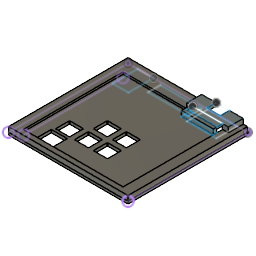
Aiwa up (Autodesk Fusion 360 design; units mm, degrees)
part number: 2026-08-31-21-16-21-827
Autodesk Fusion 360 part; units mm, degrees
note: some values were not read from the file. Chosen so that the rebuilt part matches the saved one: which bodies a step acts on. Set by a fixed rule: which sketch regions a step uses.
sketch "Sketch1" plane through (0, 0, 0) normal (0, 0, 1) x (1, 0, 0)
  line L0 (-50, 42.3306) -> (50, 42.3306)
  line L1 (50, 42.3306) -> (50, -57.6694)
  line L2 (50, -57.6694) -> (-50, -57.6694)
  line L3 (-50, -57.6694) -> (-50, 42.3306)
  line L4 (-60, 57.3306) -> (60, 57.3306)
  line L5 (60, 57.3306) -> (60, -62.6694)
  line L6 (60, -62.6694) -> (-60, -62.6694)
  line L7 (-60, -62.6694) -> (-60, 57.3306)
  dimension "d1" = 120
  dimension "d2" = 120
  dimension "d3" = 5
  dimension "d4" = 10
  dimension "d5" = 10
  dimension "d6" = 15
  constraint horizontal L0
  constraint vertical L1
  constraint horizontal L2
  constraint vertical L3
  constraint horizontal L4
  constraint vertical L5
  constraint horizontal L6
  constraint vertical L7
  measures "d1" distance of L4.start L4.end
  measures "d2" distance of L4.start L6.end
  measures "d3" distance of L2 L6
  measures "d4" distance of L3 L7
  measures "d5" distance of L1 L5
  measures "d6" distance of L0 L4
extrude "Extrude1" add sketch "Sketch1" along normal blind 3 contours L0 L1 L2 L3 makes body 1
extrude "Extrude2" add sketch "Sketch1" along normal blind 5 bodies 1
sketch "Sketch2" plane through (0, 0, 0) normal (0, 0, 1) x (1, 0, 0)
  line L0 (16.456, 54.7196) -> (-24.775, 54.7196)
  line L1 (-24.775, 54.7196) -> (-24.775, 42.3306)
  line L2 (-24.775, 42.3306) -> (16.456, 42.3306)
  line L3 (16.456, 42.3306) -> (16.456, 54.7196)
  line L4 (-60, 57.3306) -> (60, 57.3306)
  line L5 (-60, -62.6694) -> (-60, 57.3306)
  line L6 (60, 57.3306) -> (60, -62.6694)
  line L7 (-34.3292, 57.3306) -> (-50.3292, 57.3306)
  line L8 (-50.3292, 57.3306) -> (-50.3292, 32.0777)
  line L9 (-50.3292, 32.0777) -> (-34.3292, 32.0777)
  line L10 (-34.3292, 32.0777) -> (-34.3292, 57.3306)
  line L11 (-50, -57.6694) -> (-50, 42.3306)
  line L12 (20.1, 36.3376) -> (49.6, 36.3376)
  line L13 (49.6, 36.3376) -> (49.6, 57.3376)
  line L14 (49.6, 57.3376) -> (20.1, 57.3376)
  line L15 (20.1, 57.3376) -> (20.1, 36.3376)
  dimension "d11" = 41.231
  dimension "d12" = 12.389
  dimension "d14" = 35.225
  dimension "d15" = 43.544
  dimension "d18" = 16
  dimension "d72" = 29.5
  dimension "d73" = 21
  dimension "d74" = 10
  dimension "d75" = 10.4
  constraint horizontal L0
  constraint vertical L1
  constraint horizontal L2
  constraint vertical L3
  constraint horizontal L7
  constraint vertical L8
  constraint horizontal L9
  constraint vertical L10
  constraint coincident L4 L7.start
  constraint horizontal L12
  constraint vertical L13
  constraint horizontal L14
  constraint vertical L15
  measures "d11" distance of L0.start L0.end
  measures "d12" distance of L0.start L2.end
  measures "d14" distance of L1 L5
  measures "d15" distance of L3 L6
  measures "d18" distance of L7.start L7.end
  measures "d72" distance of L12.start L12.end
  measures "d73" distance of L12.start L14.end
  measures "d74" distance of L5 L11
  measures "d75" distance of L6 L13
surface "Extrude3" add extruded along (0, 0, 1) between 0 and 1.5 profiles "Sketch2" section 1 contours L4 L7 L8 L9 L10 separate body makes body 2
extrude "Extrude4" cut sketch "Sketch2" along normal blind 2.5 contours L0 L1 L2 L3 bodies 1
sketch "Sketch3" plane through (0, 0, 5) normal (0, 0, 1) x (-1, 0, 0)
  line L0 (-50, 57.6694) -> (50, 57.6694)
  line L1 (50, 57.6694) -> (50, -42.3306)
  line L2 (50, -42.3306) -> (-50, -42.3306)
  line L3 (-50, -42.3306) -> (-50, 57.6694)
  line L4 (60, 62.6694) -> (-60, 62.6694)
  line L5 (-60, 62.6694) -> (-60, -57.3306)
  line L6 (-60, -57.3306) -> (60, -57.3306)
  line L7 (60, -57.3306) -> (60, 62.6694)
  line L8 (-13.9272, -57.3306) -> (-55.7769, -57.3306)
  line L9 (-55.7769, -57.3306) -> (-55.7769, -42.3306)
  line L10 (-55.7769, -42.3306) -> (-13.9272, -42.3306)
  line L11 (-13.9272, -42.3306) -> (-13.9272, -57.3306)
  dimension "d80" = 15
  constraint horizontal L8
  constraint vertical L9
  constraint horizontal L10
  constraint vertical L11
  constraint coincident L2 L9.end
  constraint coincident L6 L8.start
  measures "d80" distance of L8.start L10.end
extrude "Extrude5" add sketch "Sketch3" along normal blind 5 contours L2 L6 L8 L9 L10 L11 bodies 1
extrude "Extrude6" cut sketch "Sketch2" along normal blind 7 contours L4 L12 L13 L15 bodies 1
extrude "Extrude7" add sketch "Sketch1" against normal blind 2.5 separate body makes body 3
extrude "Extrude8" cut sketch "Sketch2" against normal blind 2.5 contours L4 L12 L13 L15 bodies 3
extrude "Extrude9" cut sketch "Sketch2" against normal blind 2.5 contours L0 L1 L2 L3 bodies 3
extrude "Extrude10" cut sketch "Sketch2" against normal blind 2.5 contours L4 L7 L8 L9 L10 bodies 3 makes body 4 at (56.6667, 12.3306, 0)
sketch "Sketch4" plane through (0, 0, 0) normal (0, 0, 1) x (1, 0, 0)
  line L0 (38, -41.6694) -> (22, -41.6694)
  line L1 (22, -41.6694) -> (22, -56.1694)
  line L2 (22, -56.1694) -> (38, -56.1694)
  line L3 (38, -56.1694) -> (38, -41.6694)
  line L4 (50, -57.6694) -> (-50, -57.6694)
  line L5 (50, 42.3306) -> (50, -57.6694)
  dimension "d37" = 16
  dimension "d38" = 14.5
  dimension "d39" = 1.5
  dimension "d40" = 12
  constraint horizontal L0
  constraint vertical L1
  constraint horizontal L2
  constraint vertical L3
  measures "d37" distance of L0.start L0.end
  measures "d38" distance of L0.start L2.end
  measures "d39" distance of L2 L4
  measures "d40" distance of L3 L5
extrude "Extrude11" cut sketch "Sketch4" along normal blind 3 bodies 1
sketch "Sketch5" plane through (0, 0, 0) normal (0, 0, -1) x (1, 0, 0)
  line L0 (22, 56.1694) -> (38, 56.1694)
  line L1 (38, 56.1694) -> (38, 41.6694)
  line L2 (38, 41.6694) -> (22, 41.6694)
  line L3 (22, 41.6694) -> (22, 56.1694)
  line L4 (49.6, -57.3306) -> (60, -57.3306)
  line L5 (60, -57.3306) -> (60, 62.6694)
  line L6 (60, 62.6694) -> (-60, 62.6694)
  line L7 (-60, 62.6694) -> (-60, -57.3306)
  line L8 (-60, -57.3306) -> (20.1, -57.3306)
  line L9 (-24.775, -42.3306) -> (16.456, -42.3306)
  line L10 (16.456, -42.3306) -> (16.456, -54.7196)
  line L11 (16.456, -54.7196) -> (-24.775, -54.7196)
  line L12 (-24.775, -54.7196) -> (-24.775, -42.3306)
  line L13 (18.153, 22.4292) -> (-0.897, 22.4292)
  line L14 (-0.897, 22.4292) -> (-0.897, 41.4792)
  line L15 (-0.897, 41.4792) -> (18.153, 41.4792)
  line L16 (18.153, 41.4792) -> (18.153, 22.4292)
  line L17 (50, -42.3306) -> (50, 57.6694)
  line L18 (2.0861, 38.928) -> (15.0861, 38.928)
  line L19 (2.0861, 24.928) -> (15.0861, 24.928)
  line L20 (1.5861, 38.428) -> (1.5861, 25.428)
  line L21 (15.5861, 38.428) -> (15.5861, 25.428)
  arc A0 (2.0861, 38.928) -> (1.5861, 38.428) centre (2.0861, 38.428) ccw
  arc A1 (15.5861, 38.428) -> (15.0861, 38.928) centre (15.0861, 38.428) ccw
  arc A2 (1.5861, 25.428) -> (2.0861, 24.928) centre (2.0861, 25.428) ccw
  arc A3 (15.0861, 24.928) -> (15.5861, 25.428) centre (15.0861, 25.428) ccw
  line L22 (-0.9389, 22.403) -> (18.1111, 22.403)
  line L23 (-0.9389, 41.453) -> (18.1111, 41.453)
  line L24 (-0.9389, 22.403) -> (-0.9389, 41.453)
  line L25 (18.1111, 22.403) -> (18.1111, 41.453)
  line L26 (-16.9175, 38.9647) -> (-3.9175, 38.9647)
  line L27 (-16.9175, 24.9647) -> (-3.9175, 24.9647)
  line L28 (-17.4175, 38.4647) -> (-17.4175, 25.4647)
  line L29 (-3.4175, 38.4647) -> (-3.4175, 25.4647)
  arc A4 (-16.9175, 38.9647) -> (-17.4175, 38.4647) centre (-16.9175, 38.4647) ccw
  arc A5 (-3.4175, 38.4647) -> (-3.9175, 38.9647) centre (-3.9175, 38.4647) ccw
  arc A6 (-17.4175, 25.4647) -> (-16.9175, 24.9647) centre (-16.9175, 25.4647) ccw
  arc A7 (-3.9175, 24.9647) -> (-3.4175, 25.4647) centre (-3.9175, 25.4647) ccw
  line L30 (-19.9425, 22.4397) -> (-0.8925, 22.4397)
  line L31 (-19.9425, 41.4897) -> (-0.8925, 41.4897)
  line L32 (-19.9425, 22.4397) -> (-19.9425, 41.4897)
  line L33 (-0.8925, 22.4397) -> (-0.8925, 41.4897)
  line L34 (-35.9551, 38.9464) -> (-22.9551, 38.9464)
  line L35 (-35.9551, 24.9464) -> (-22.9551, 24.9464)
  line L36 (-36.4551, 38.4464) -> (-36.4551, 25.4464)
  line L37 (-22.4551, 38.4464) -> (-22.4551, 25.4464)
  arc A8 (-35.9551, 38.9464) -> (-36.4551, 38.4464) centre (-35.9551, 38.4464) ccw
  arc A9 (-22.4551, 38.4464) -> (-22.9551, 38.9464) centre (-22.9551, 38.4464) ccw
  arc A10 (-36.4551, 25.4464) -> (-35.9551, 24.9464) centre (-35.9551, 25.4464) ccw
  arc A11 (-22.9551, 24.9464) -> (-22.4551, 25.4464) centre (-22.9551, 25.4464) ccw
  line L38 (-38.9801, 22.4214) -> (-19.9301, 22.4214)
  line L39 (-38.9801, 41.4714) -> (-19.9301, 41.4714)
  line L40 (-38.9801, 22.4214) -> (-38.9801, 41.4714)
  line L41 (-19.9301, 22.4214) -> (-19.9301, 41.4714)
  line L42 (2.0843, 19.8957) -> (15.0843, 19.8957)
  line L43 (2.0843, 5.8957) -> (15.0843, 5.8957)
  line L44 (1.5843, 19.3957) -> (1.5843, 6.3957)
  line L45 (15.5843, 19.3957) -> (15.5843, 6.3957)
  arc A12 (2.0843, 19.8957) -> (1.5843, 19.3957) centre (2.0843, 19.3957) ccw
  arc A13 (15.5843, 19.3957) -> (15.0843, 19.8957) centre (15.0843, 19.3957) ccw
  arc A14 (1.5843, 6.3957) -> (2.0843, 5.8957) centre (2.0843, 6.3957) ccw
  arc A15 (15.0843, 5.8957) -> (15.5843, 6.3957) centre (15.0843, 6.3957) ccw
  line L46 (-0.9407, 3.3707) -> (18.1093, 3.3707)
  line L47 (-0.9407, 22.4207) -> (18.1093, 22.4207)
  line L48 (-0.9407, 3.3707) -> (-0.9407, 22.4207)
  line L49 (18.1093, 3.3707) -> (18.1093, 22.4207)
  line L50 (-16.977, 19.904) -> (-3.977, 19.904)
  line L51 (-16.977, 5.904) -> (-3.977, 5.904)
  line L52 (-17.477, 19.404) -> (-17.477, 6.404)
  line L53 (-3.477, 19.404) -> (-3.477, 6.404)
  arc A16 (-16.977, 19.904) -> (-17.477, 19.404) centre (-16.977, 19.404) ccw
  arc A17 (-3.477, 19.404) -> (-3.977, 19.904) centre (-3.977, 19.404) ccw
  arc A18 (-17.477, 6.404) -> (-16.977, 5.904) centre (-16.977, 6.404) ccw
  arc A19 (-3.977, 5.904) -> (-3.477, 6.404) centre (-3.977, 6.404) ccw
  line L54 (-20.002, 3.379) -> (-0.952, 3.379)
  line L55 (-20.002, 22.429) -> (-0.952, 22.429)
  line L56 (-20.002, 3.379) -> (-20.002, 22.429)
  line L57 (-0.952, 3.379) -> (-0.952, 22.429)
  line L58 (-50, 57.6694) -> (-50, -42.3306)
  line L59 (-22, 41.6694) -> (-38, 41.6694)
  line L60 (-38, 41.6694) -> (-38, 56.1694)
  line L61 (-38, 56.1694) -> (-22, 56.1694)
  line L62 (-22, 56.1694) -> (-22, 41.6694)
  line L63 (50, 57.6694) -> (-50, 57.6694)
  line L64 (49.6, -36.3376) -> (49.6, -57.3306)
  line L65 (20.1, -57.3306) -> (20.1, -36.3376)
  line L66 (20.1, -36.3376) -> (49.6, -36.3376)
  dimension "d43" = 19.05
  dimension "d44" = 19.05
  dimension "d57" = 72
  dimension "d58" = 12
  dimension "d61" = 16
  dimension "d62" = 14.5
  dimension "d63" = 16
  dimension "d64" = 14.5
  dimension "d65" = 1.5
  dimension "d66" = 12
  dimension "d68" = 11.0199
  constraint horizontal L13
  constraint vertical L14
  constraint horizontal L15
  constraint vertical L16
  constraint horizontal L59
  constraint vertical L60
  constraint horizontal L61
  constraint vertical L62
  measures "d43" distance of L13.start L13.end
  measures "d44" distance of L13.start L15.end
  measures "d57" distance of L3 L58
  measures "d58" distance of L1 L17
  measures "d61" distance of L0.start L0.end
  measures "d62" distance of L0.start L2.end
  measures "d63" distance of L59.start L59.end
  measures "d64" distance of L59.start L61.end
  measures "d65" distance of L61 L63
  measures "d66" distance of L58 L60
  measures "d68" distance of L40 L58
extrude "Extrude12" cut sketch "Sketch5" against normal blind 3 contours L18 L19 L20 L21 A0 A1 A2 A3 bodies 1
extrude "Extrude13" cut sketch "Sketch5" against normal blind 3 contours L26 L27 L28 L29 A4 A5 A6 A7 bodies 1
extrude "Extrude14" cut sketch "Sketch5" against normal blind 3 contours L34 L35 L36 L37 A8 A9 A10 A11 bodies 1
extrude "Extrude15" cut sketch "Sketch5" against normal blind 3 contours L50 L51 L52 L53 A16 A17 A18 A19 bodies 1
extrude "Extrude16" cut sketch "Sketch5" against normal blind 3 contours L42 L43 L44 L45 A12 A13 A14 A15 bodies 1
extrude "Extrude17" add sketch "Sketch5" against normal blind 3 contours L0 L1 L2 L3 bodies 1
extrude "Extrude18" cut sketch "Sketch5" against normal blind 3 contours L59 L60 L61 L62 bodies 1
extrude "Extrude19" add 1 faces at (56.6667, 12.3306, -2.5) along direction (0, 0, -1) blind 2.5 on bodies 4 bodies 4
extrude "Extrude20" cut 1 faces at (56.6667, 12.3306, -5) along direction (0, 0, 1) blind 2.5 on bodies 4 bodies 4
sketch "Sketch6" plane through (0, 0, 5) normal (0, 0, 1) x (-1, 0, 0)
  line L0 (-50, -33) -> (-17.9437, -33)
  line L1 (-17.9437, -33) -> (-17.9437, -36.4428)
  line L2 (-17.9437, -36.4428) -> (-50, -36.4428)
  line L3 (-50, -36.4428) -> (-50, -33)
  line L4 (-20.42, -36.4428) -> (-17.9437, -36.4428)
  line L5 (-17.9437, -36.4428) -> (-17.9437, -42.305)
  line L6 (-17.9437, -42.305) -> (-20.42, -42.305)
  line L7 (-20.42, -42.305) -> (-20.42, -36.4428)
  constraint horizontal L0
  constraint vertical L1
  constraint horizontal L2
  constraint vertical L3
  constraint horizontal L4
  constraint vertical L5
  constraint horizontal L6
  constraint vertical L7
  constraint coincident L2 L4.start
extrude "Extrude21" add sketch "Sketch6" along normal blind 5 separate body contours L0 L1 L2 L3 L4 makes body 5
extrude "Extrude22" add sketch "Sketch6" along normal blind 5 contours L2 L4 L5 L6 L7 bodies 5
sketch "Sketch7" plane through (0, 0, 10) normal (0, 0, 1) x (-1, 0, 0)
  line L0 (-13.9272, -42.3306) -> (-55.7769, -42.3306)
  line L1 (-55.7769, -42.3306) -> (-55.7769, -57.3306)
  line L2 (-55.7769, -57.3306) -> (-13.9272, -57.3306)
  line L3 (-13.9272, -57.3306) -> (-13.9272, -42.3306)
  line L4 (-50.001, -36.4538) -> (-19.85, -36.4538)
  line L5 (-19.85, -36.4538) -> (-19.85, -42.3306)
  line L6 (-19.85, -42.3306) -> (-50.001, -42.3306)
  line L7 (-50.001, -42.3306) -> (-50.001, -36.4538)
  line L8 (-42, -48) -> (-28.5728, -48)
  line L9 (-28.5728, -48) -> (-28.5728, -57.3306)
  line L10 (-28.5728, -57.3306) -> (-42, -57.3306)
  line L11 (-42, -57.3306) -> (-42, -48)
  constraint horizontal L4
  constraint vertical L5
  constraint horizontal L6
  constraint vertical L7
  constraint coincident L0 L5.end
  constraint horizontal L8
  constraint vertical L9
  constraint horizontal L10
  constraint vertical L11
  constraint coincident L2 L9.end
extrude "Extrude23" add sketch "Sketch7" against normal blind 2 contours L0 L4 L5 L6 L7 bodies 1
extrude "Extrude24" cut sketch "Sketch7" against normal blind 3 contours L2 L8 L9 L10 L11 bodies 1
